Autodesk Inventor part; units mm, degrees
(part 6 of 6)
  line L4439 (-10.0121, 28.4168) -> (-10.0047, 28.6447)
  line L4440 (-10.0047, 28.6447) -> (-9.9918, 28.8863)
  line L4441 (-9.9918, 28.8863) -> (-9.973, 29.1388)
  line L4442 (-9.973, 29.1388) -> (-9.9523, 29.359)
  arc A136 (-9.2052, 29.6018) -> (-9.9523, 29.359) centre (0, 0) ccw
  line L4443 (-9.2052, 29.6018) -> (-9.059, 29.4358)
  line L4444 (-9.059, 29.4358) -> (-8.8954, 29.2425)
  line L4445 (-8.8954, 29.2425) -> (-8.7429, 29.0547)
  line L4446 (-8.7429, 29.0547) -> (-8.603, 28.8746)
  line L4447 (-8.603, 28.8746) -> (-8.4737, 28.7009)
  line L4448 (-8.4737, 28.7009) -> (-8.3547, 28.5338)
  line L4449 (-8.3547, 28.5338) -> (-8.2472, 28.3759)
  line L4450 (-8.2472, 28.3759) -> (-8.1494, 28.2257)
  line L4451 (-8.1494, 28.2257) -> (-7.9652, 27.9266)
  line L4452 (-7.9652, 27.9266) -> (-7.9351, 27.8907)
  line L4453 (-7.9351, 27.8907) -> (-7.9073, 27.8683)
  line L4454 (-7.9073, 27.8683) -> (-7.8823, 27.8592)
  line L4455 (-7.8823, 27.8592) -> (-7.8657, 27.861)
  line L4456 (-7.8657, 27.861) -> (-7.4928, 27.9636)
  line L4457 (-7.4928, 27.9636) -> (-7.1186, 28.0612)
  line L4458 (-7.1186, 28.0612) -> (-7.1033, 28.0679)
  line L4459 (-7.1033, 28.0679) -> (-7.0862, 28.0883)
  line L4460 (-7.0862, 28.0883) -> (-7.0733, 28.1216)
  line L4461 (-7.0733, 28.1216) -> (-7.0652, 28.1677)
  line L4462 (-7.0652, 28.1677) -> (-7.0553, 28.5189)
  line L4463 (-7.0553, 28.5189) -> (-7.0457, 28.6979)
  line L4464 (-7.0457, 28.6979) -> (-7.0315, 28.8883)
  line L4465 (-7.0315, 28.8883) -> (-7.012, 29.0926)
  line L4466 (-7.012, 29.0926) -> (-6.9869, 29.3077)
  line L4467 (-6.9869, 29.3077) -> (-6.9557, 29.5336)
  line L4468 (-6.9557, 29.5336) -> (-6.9177, 29.7725)
  line L4469 (-6.9177, 29.7725) -> (-6.8726, 30.0216)
  line L4470 (-6.8726, 30.0216) -> (-6.829, 30.2385)
  arc A137 (-6.0605, 30.4018) -> (-6.829, 30.2385) centre (0, 0) ccw
  line L4471 (-6.0605, 30.4018) -> (-5.9325, 30.2214)
  line L4472 (-5.9325, 30.2214) -> (-5.79, 30.0122)
  line L4473 (-5.79, 30.0122) -> (-5.658, 29.8094)
  line L4474 (-5.658, 29.8094) -> (-5.5376, 29.6157)
  line L4475 (-5.5376, 29.6157) -> (-5.4272, 29.4294)
  line L4476 (-5.4272, 29.4294) -> (-5.3263, 29.2508)
  line L4477 (-5.3263, 29.2508) -> (-5.2359, 29.0826)
  line L4478 (-5.2359, 29.0826) -> (-5.1544, 28.9229)
  line L4479 (-5.1544, 28.9229) -> (-5.0025, 28.6062)
  line L4480 (-5.0025, 28.6062) -> (-4.9763, 28.5674)
  line L4481 (-4.9763, 28.5674) -> (-4.951, 28.5421)
  line L4482 (-4.951, 28.5421) -> (-4.927, 28.5305)
  line L4483 (-4.927, 28.5305) -> (-4.9104, 28.5306)
  line L4484 (-4.9104, 28.5306) -> (-4.5288, 28.5936)
  line L4485 (-4.5288, 28.5936) -> (-4.1464, 28.6516)
  line L4486 (-4.1464, 28.6516) -> (-4.1305, 28.6567)
  line L4487 (-4.1305, 28.6567) -> (-4.1114, 28.6751)
  line L4488 (-4.1114, 28.6751) -> (-4.0951, 28.7069)
  line L4489 (-4.0951, 28.7069) -> (-4.0822, 28.7519)
  line L4490 (-4.0822, 28.7519) -> (-4.0356, 29.1001)
  line L4491 (-4.0356, 29.1001) -> (-4.0074, 29.2771)
  line L4492 (-4.0074, 29.2771) -> (-3.9734, 29.465)
  line L4493 (-3.9734, 29.465) -> (-3.9326, 29.6661)
  line L4494 (-3.9326, 29.6661) -> (-3.8852, 29.8774)
  line L4495 (-3.8852, 29.8774) -> (-3.8305, 30.0989)
  line L4496 (-3.8305, 30.0989) -> (-3.7677, 30.3325)
  line L4497 (-3.7677, 30.3325) -> (-3.6968, 30.5755)
  line L4498 (-3.6968, 30.5755) -> (-3.6308, 30.7866)
  arc A138 (-2.8495, 30.8688) -> (-3.6308, 30.7866) centre (0, 0) ccw
  line L4499 (-2.8495, 30.8688) -> (-2.741, 30.676)
  line L4500 (-2.741, 30.676) -> (-2.6211, 30.453)
  line L4501 (-2.6211, 30.453) -> (-2.5111, 30.2376)
  line L4502 (-2.5111, 30.2376) -> (-2.4116, 30.0323)
  line L4503 (-2.4116, 30.0323) -> (-2.3213, 29.8355)
  line L4504 (-2.3213, 29.8355) -> (-2.2396, 29.6473)
  line L4505 (-2.2396, 29.6473) -> (-2.1673, 29.4705)
  line L4506 (-2.1673, 29.4705) -> (-2.1029, 29.3033)
  line L4507 (-2.1029, 29.3033) -> (-1.9849, 28.9724)
  line L4508 (-1.9849, 28.9724) -> (-1.9629, 28.931)
  line L4509 (-1.9629, 28.931) -> (-1.9404, 28.9033)
  line L4510 (-1.9404, 28.9033) -> (-1.9178, 28.8892)
  line L4511 (-1.9178, 28.8892) -> (-1.9012, 28.8876)
  line L4512 (-1.9012, 28.8876) -> (-1.5151, 28.9103)
  line L4513 (-1.5151, 28.9103) -> (-1.1288, 28.9281)
  line L4514 (-1.1288, 28.9281) -> (-1.1124, 28.9314)
  line L4515 (-1.1124, 28.9314) -> (-1.0915, 28.9478)
  line L4516 (-1.0915, 28.9478) -> (-1.0719, 28.9777)
  line L4517 (-1.0719, 28.9777) -> (-1.0544, 29.0211)
  line L4518 (-1.0544, 29.0211) -> (-0.9717, 29.3626)
  line L4519 (-0.9717, 29.3626) -> (-0.9251, 29.5356)
  line L4520 (-0.9251, 29.5356) -> (-0.8717, 29.719)
  line L4521 (-0.8717, 29.719) -> (-0.8101, 29.9147)
  line L4522 (-0.8101, 29.9147) -> (-0.7408, 30.1199)
  line L4523 (-0.7408, 30.1199) -> (-0.6634, 30.3344)
  line L4524 (-0.6634, 30.3344) -> (-0.5765, 30.5601)
  line L4525 (-0.5765, 30.5601) -> (-0.4805, 30.7945)
  line L4526 (-0.4805, 30.7945) -> (-0.3928, 30.9975)
  arc A139 (0.3928, 30.9975) -> (-0.3928, 30.9975) centre (0, 0) ccw
  line L4527 (0.3928, 30.9975) -> (0.4805, 30.7945)
  line L4528 (0.4805, 30.7945) -> (0.5765, 30.5601)
  line L4529 (0.5765, 30.5601) -> (0.6634, 30.3344)
  line L4530 (0.6634, 30.3344) -> (0.7408, 30.1199)
  line L4531 (0.7408, 30.1199) -> (0.8101, 29.9147)
  line L4532 (0.8101, 29.9147) -> (0.8717, 29.719)
  line L4533 (0.8717, 29.719) -> (0.9251, 29.5356)
  line L4534 (0.9251, 29.5356) -> (0.9717, 29.3626)
  line L4535 (0.9717, 29.3626) -> (1.0544, 29.0211)
  line L4536 (1.0544, 29.0211) -> (1.0719, 28.9777)
  line L4537 (1.0719, 28.9777) -> (1.0915, 28.9478)
  line L4538 (1.0915, 28.9478) -> (1.1124, 28.9314)
  line L4539 (1.1124, 28.9314) -> (1.1288, 28.9281)
  line L4540 (1.1288, 28.9281) -> (1.5151, 28.9103)
  line L4541 (1.5151, 28.9103) -> (1.9012, 28.8876)
  line L4542 (1.9012, 28.8876) -> (1.9178, 28.8892)
  line L4543 (1.9178, 28.8892) -> (1.9404, 28.9033)
  line L4544 (1.9404, 28.9033) -> (1.9629, 28.931)
  line L4545 (1.9629, 28.931) -> (1.9849, 28.9724)
  line L4546 (1.9849, 28.9724) -> (2.1029, 29.3033)
  line L4547 (2.1029, 29.3033) -> (2.1673, 29.4705)
  line L4548 (2.1673, 29.4705) -> (2.2396, 29.6473)
  line L4549 (2.2396, 29.6473) -> (2.3213, 29.8355)
  line L4550 (2.3213, 29.8355) -> (2.4116, 30.0323)
  line L4551 (2.4116, 30.0323) -> (2.5111, 30.2376)
  line L4552 (2.5111, 30.2376) -> (2.6211, 30.453)
  line L4553 (2.6211, 30.453) -> (2.741, 30.676)
  line L4554 (2.741, 30.676) -> (2.8495, 30.8688)
  arc A140 (3.6308, 30.7866) -> (2.8495, 30.8688) centre (0, 0) ccw
  line L4555 (3.6308, 30.7866) -> (3.6968, 30.5755)
  line L4556 (3.6968, 30.5755) -> (3.7677, 30.3325)
  line L4557 (3.7677, 30.3325) -> (3.8305, 30.0989)
  line L4558 (3.8305, 30.0989) -> (3.8852, 29.8774)
  line L4559 (3.8852, 29.8774) -> (3.9326, 29.6661)
  line L4560 (3.9326, 29.6661) -> (3.9734, 29.465)
  line L4561 (3.9734, 29.465) -> (4.0074, 29.2771)
  line L4562 (4.0074, 29.2771) -> (4.0356, 29.1001)
  line L4563 (4.0356, 29.1001) -> (4.0822, 28.7519)
  line L4564 (4.0822, 28.7519) -> (4.0951, 28.7069)
  line L4565 (4.0951, 28.7069) -> (4.1114, 28.6751)
  line L4566 (4.1114, 28.6751) -> (4.1305, 28.6567)
  line L4567 (4.1305, 28.6567) -> (4.1464, 28.6516)
  line L4568 (4.1464, 28.6516) -> (4.5288, 28.5936)
  line L4569 (4.5288, 28.5936) -> (4.9104, 28.5306)
  line L4570 (4.9104, 28.5306) -> (4.927, 28.5305)
  line L4571 (4.927, 28.5305) -> (4.951, 28.5421)
  line L4572 (4.951, 28.5421) -> (4.9763, 28.5674)
  line L4573 (4.9763, 28.5674) -> (5.0025, 28.6062)
  line L4574 (5.0025, 28.6062) -> (5.1544, 28.9229)
  line L4575 (5.1544, 28.9229) -> (5.2359, 29.0826)
  line L4576 (5.2359, 29.0826) -> (5.3263, 29.2508)
  line L4577 (5.3263, 29.2508) -> (5.4272, 29.4294)
  line L4578 (5.4272, 29.4294) -> (5.5376, 29.6157)
  line L4579 (5.5376, 29.6157) -> (5.658, 29.8094)
  line L4580 (5.658, 29.8094) -> (5.79, 30.0122)
  line L4581 (5.79, 30.0122) -> (5.9325, 30.2214)
  line L4582 (5.9325, 30.2214) -> (6.0605, 30.4018)
  arc A141 (6.829, 30.2385) -> (6.0605, 30.4018) centre (0, 0) ccw
  line L4583 (6.829, 30.2385) -> (6.8726, 30.0216)
  line L4584 (6.8726, 30.0216) -> (6.9177, 29.7725)
  line L4585 (6.9177, 29.7725) -> (6.9557, 29.5336)
  line L4586 (6.9557, 29.5336) -> (6.9869, 29.3077)
  line L4587 (6.9869, 29.3077) -> (7.012, 29.0926)
  line L4588 (7.012, 29.0926) -> (7.0315, 28.8883)
  line L4589 (7.0315, 28.8883) -> (7.0457, 28.6979)
  line L4590 (7.0457, 28.6979) -> (7.0553, 28.5189)
  line L4591 (7.0553, 28.5189) -> (7.0652, 28.1677)
  line L4592 (7.0652, 28.1677) -> (7.0733, 28.1216)
  line L4593 (7.0733, 28.1216) -> (7.0862, 28.0883)
  line L4594 (7.0862, 28.0883) -> (7.1033, 28.0679)
  line L4595 (7.1033, 28.0679) -> (7.1186, 28.0612)
  line L4596 (7.1186, 28.0612) -> (7.4928, 27.9636)
  line L4597 (7.4928, 27.9636) -> (7.8657, 27.861)
  line L4598 (7.8657, 27.861) -> (7.8823, 27.8592)
  line L4599 (7.8823, 27.8592) -> (7.9073, 27.8683)
  line L4600 (7.9073, 27.8683) -> (7.9351, 27.8907)
  line L4601 (7.9351, 27.8907) -> (7.9652, 27.9266)
  line L4602 (7.9652, 27.9266) -> (8.1494, 28.2257)
  line L4603 (8.1494, 28.2257) -> (8.2472, 28.3759)
  line L4604 (8.2472, 28.3759) -> (8.3547, 28.5338)
  line L4605 (8.3547, 28.5338) -> (8.4737, 28.7009)
  line L4606 (8.4737, 28.7009) -> (8.603, 28.8746)
  line L4607 (8.603, 28.8746) -> (8.7429, 29.0547)
  line L4608 (8.7429, 29.0547) -> (8.8954, 29.2425)
  line L4609 (8.8954, 29.2425) -> (9.059, 29.4358)
  line L4610 (9.059, 29.4358) -> (9.2052, 29.6018)
  arc A142 (9.9523, 29.359) -> (9.2052, 29.6018) centre (0, 0) ccw
  line L4611 (9.9523, 29.359) -> (9.973, 29.1388)
  line L4612 (9.973, 29.1388) -> (9.9918, 28.8863)
  line L4613 (9.9918, 28.8863) -> (10.0047, 28.6447)
  line L4614 (10.0047, 28.6447) -> (10.0121, 28.4168)
  line L4615 (10.0121, 28.4168) -> (10.0146, 28.2002)
  line L4616 (10.0146, 28.2002) -> (10.0127, 27.995)
  line L4617 (10.0127, 27.995) -> (10.0069, 27.8042)
  line L4618 (10.0069, 27.8042) -> (9.9977, 27.6252)
  line L4619 (9.9977, 27.6252) -> (9.9708, 27.2749)
  line L4620 (9.9708, 27.2749) -> (9.9741, 27.2282)
  line L4621 (9.9741, 27.2282) -> (9.9834, 27.1937)
  line L4622 (9.9834, 27.1937) -> (9.9983, 27.1717)
  line L4623 (9.9983, 27.1717) -> (10.0128, 27.1634)
  line L4624 (10.0128, 27.1634) -> (10.3748, 27.0272)
  line L4625 (10.3748, 27.0272) -> (10.7349, 26.8862)
  line L4626 (10.7349, 26.8862) -> (10.7512, 26.8826)
  line L4627 (10.7512, 26.8826) -> (10.777, 26.8891)
  line L4628 (10.777, 26.8891) -> (10.807, 26.9085)
  line L4629 (10.807, 26.9085) -> (10.8407, 26.941)
  line L4630 (10.8407, 26.941) -> (11.0551, 27.2193)
  line L4631 (11.0551, 27.2193) -> (11.1681, 27.3584)
  line L4632 (11.1681, 27.3584) -> (11.2915, 27.5042)
  line L4633 (11.2915, 27.5042) -> (11.4273, 27.6579)
  line L4634 (11.4273, 27.6579) -> (11.5741, 27.8172)
  line L4635 (11.5741, 27.8172) -> (11.7321, 27.9817)
  line L4636 (11.7321, 27.9817) -> (11.9033, 28.1525)
  line L4637 (11.9033, 28.1525) -> (12.0862, 28.3276)
  line L4638 (12.0862, 28.3276) -> (12.249, 28.4774)
  arc A143 (12.9667, 28.1579) -> (12.249, 28.4774) centre (0, 0) ccw
  line L4639 (12.9667, 28.1579) -> (12.9642, 27.9367)
  line L4640 (12.9642, 27.9367) -> (12.9565, 27.6836)
  line L4641 (12.9565, 27.6836) -> (12.9441, 27.442)
  line L4642 (12.9441, 27.442) -> (12.9276, 27.2145)
  line L4643 (12.9276, 27.2145) -> (12.9075, 26.9989)
  line L4644 (12.9075, 26.9989) -> (12.8841, 26.7951)
  line L4645 (12.8841, 26.7951) -> (12.8584, 26.6059)
  line L4646 (12.8584, 26.6059) -> (12.8305, 26.4288)
  line L4647 (12.8305, 26.4288) -> (12.7672, 26.0833)
  line L4648 (12.7672, 26.0833) -> (12.7656, 26.0365)
  line L4649 (12.7656, 26.0365) -> (12.7712, 26.0012)
  line L4650 (12.7712, 26.0012) -> (12.7837, 25.9777)
  line L4651 (12.7837, 25.9777) -> (12.7973, 25.968)
  line L4652 (12.7973, 25.968) -> (13.143, 25.7946)
  line L4653 (13.143, 25.7946) -> (13.4865, 25.6168)
  line L4654 (13.4865, 25.6168) -> (13.5023, 25.6116)
  line L4655 (13.5023, 25.6116) -> (13.5287, 25.6153)
  line L4656 (13.5287, 25.6153) -> (13.5605, 25.6314)
  line L4657 (13.5605, 25.6314) -> (13.5974, 25.6603)
  line L4658 (13.5974, 25.6603) -> (13.8398, 25.9146)
  line L4659 (13.8398, 25.9146) -> (13.9666, 26.0412)
  line L4660 (13.9666, 26.0412) -> (14.1046, 26.1732)
  line L4661 (14.1046, 26.1732) -> (14.2558, 26.312)
  line L4662 (14.2558, 26.312) -> (14.4184, 26.455)
  line L4663 (14.4184, 26.455) -> (14.5927, 26.602)
  line L4664 (14.5927, 26.602) -> (14.7808, 26.7541)
  line L4665 (14.7808, 26.7541) -> (14.9811, 26.9091)
  line L4666 (14.9811, 26.9091) -> (15.1586, 27.041)
  arc A144 (15.8389, 26.6482) -> (15.1586, 27.041) centre (0, 0) ccw
  line L4667 (15.8389, 26.6482) -> (15.8134, 26.4285)
  line L4668 (15.8134, 26.4285) -> (15.7793, 26.1776)
  line L4669 (15.7793, 26.1776) -> (15.7417, 25.9387)
  line L4670 (15.7417, 25.9387) -> (15.7015, 25.7142)
  line L4671 (15.7015, 25.7142) -> (15.6589, 25.5018)
  line L4672 (15.6589, 25.5018) -> (15.6144, 25.3015)
  line L4673 (15.6144, 25.3015) -> (15.569, 25.1161)
  line L4674 (15.569, 25.1161) -> (15.5228, 24.9429)
  line L4675 (15.5228, 24.9429) -> (15.4237, 24.6058)
  line L4676 (15.4237, 24.6058) -> (15.4172, 24.5595)
  line L4677 (15.4172, 24.5595) -> (15.4191, 24.5238)
  line L4678 (15.4191, 24.5238) -> (15.4291, 24.4991)
  line L4679 (15.4291, 24.4991) -> (15.4416, 24.488)
  line L4680 (15.4416, 24.488) -> (15.7673, 24.2795)
  line L4681 (15.7673, 24.2795) -> (16.0903, 24.0668)
  line L4682 (16.0903, 24.0668) -> (16.1055, 24.0599)
  line L4683 (16.1055, 24.0599) -> (16.1321, 24.0608)
  line L4684 (16.1321, 24.0608) -> (16.1655, 24.0735)
  line L4685 (16.1655, 24.0735) -> (16.2052, 24.0984)
  line L4686 (16.2052, 24.0984) -> (16.4728, 24.326)
  line L4687 (16.4728, 24.326) -> (16.6122, 24.4386)
  line L4688 (16.6122, 24.4386) -> (16.7632, 24.5555)
  line L4689 (16.7632, 24.5555) -> (16.928, 24.6777)
  line L4690 (16.928, 24.6777) -> (17.1047, 24.8029)
  line L4691 (17.1047, 24.8029) -> (17.2934, 24.931)
  line L4692 (17.2934, 24.931) -> (17.4964, 25.0625)
  line L4693 (17.4964, 25.0625) -> (17.7118, 25.1957)
  line L4694 (17.7118, 25.1957) -> (17.9021, 25.3084)
  arc A145 (18.5377, 24.8466) -> (17.9021, 25.3084) centre (0, 0) ccw
  line L4695 (18.5377, 24.8466) -> (18.4893, 24.6308)
  line L4696 (18.4893, 24.6308) -> (18.4292, 24.3848)
  line L4697 (18.4292, 24.3848) -> (18.3668, 24.1511)
  line L4698 (18.3668, 24.1511) -> (18.3034, 23.932)
  line L4699 (18.3034, 23.932) -> (18.2388, 23.7253)
  line L4700 (18.2388, 23.7253) -> (18.1736, 23.5308)
  line L4701 (18.1736, 23.5308) -> (18.1091, 23.3511)
  line L4702 (18.1091, 23.3511) -> (18.045, 23.1837)
  line L4703 (18.045, 23.1837) -> (17.9112, 22.8588)
  line L4704 (17.9112, 22.8588) -> (17.8999, 22.8134)
  line L4705 (17.8999, 22.8134) -> (17.8981, 22.7777)
  line L4706 (17.8981, 22.7777) -> (17.9055, 22.7521)
  line L4707 (17.9055, 22.7521) -> (17.9167, 22.7398)
  line L4708 (17.9167, 22.7398) -> (18.2188, 22.4984)
  line L4709 (18.2188, 22.4984) -> (18.5178, 22.2531)
  line L4710 (18.5178, 22.2531) -> (18.5322, 22.2446)
  line L4711 (18.5322, 22.2446) -> (18.5587, 22.2427)
  line L4712 (18.5587, 22.2427) -> (18.5933, 22.2519)
  line L4713 (18.5933, 22.2519) -> (18.6353, 22.2724)
  line L4714 (18.6353, 22.2724) -> (18.9253, 22.4708)
  line L4715 (18.9253, 22.4708) -> (19.0757, 22.5683)
  line L4716 (19.0757, 22.5683) -> (19.2381, 22.6688)
  line L4717 (19.2381, 22.6688) -> (19.4148, 22.773)
  line L4718 (19.4148, 22.773) -> (19.6036, 22.8791)
  line L4719 (19.6036, 22.8791) -> (19.8047, 22.9867)
  line L4720 (19.8047, 22.9867) -> (20.0203, 23.0963)
  line L4721 (20.0203, 23.0963) -> (20.2484, 23.2063)
  line L4722 (20.2484, 23.2063) -> (20.4495, 23.2985)
  arc A146 (21.0333, 22.7728) -> (20.4495, 23.2985) centre (0, 0) ccw
  line L4723 (21.0333, 22.7728) -> (20.9626, 22.5632)
  line L4724 (20.9626, 22.5632) -> (20.8771, 22.3249)
  line L4725 (20.8771, 22.3249) -> (20.7906, 22.099)
  line L4726 (20.7906, 22.099) -> (20.7047, 21.8877)
  line L4727 (20.7047, 21.8877) -> (20.6189, 21.6889)
  line L4728 (20.6189, 21.6889) -> (20.5336, 21.5022)
  line L4729 (20.5336, 21.5022) -> (20.4507, 21.3302)
  line L4730 (20.4507, 21.3302) -> (20.3695, 21.1705)
  line L4731 (20.3695, 21.1705) -> (20.2025, 20.8614)
  line L4732 (20.2025, 20.8614) -> (20.1865, 20.8174)
  line L4733 (20.1865, 20.8174) -> (20.181, 20.7821)
  line L4734 (20.181, 20.7821) -> (20.1856, 20.7559)
  line L4735 (20.1856, 20.7559) -> (20.1955, 20.7424)
  line L4736 (20.1955, 20.7424) -> (20.4707, 20.4707)
  line L4737 (20.4707, 20.4707) -> (20.7424, 20.1955)
  line L4738 (20.7424, 20.1955) -> (20.7559, 20.1856)
  line L4739 (20.7559, 20.1856) -> (20.7821, 20.181)
  line L4740 (20.7821, 20.181) -> (20.8174, 20.1865)
  line L4741 (20.8174, 20.1865) -> (20.8614, 20.2025)
  line L4742 (20.8614, 20.2025) -> (21.1705, 20.3695)
  line L4743 (21.1705, 20.3695) -> (21.3302, 20.4507)
  line L4744 (21.3302, 20.4507) -> (21.5022, 20.5336)
  line L4745 (21.5022, 20.5336) -> (21.6889, 20.6189)
  line L4746 (21.6889, 20.6189) -> (21.8877, 20.7047)
  line L4747 (21.8877, 20.7047) -> (22.099, 20.7906)
  line L4748 (22.099, 20.7906) -> (22.3249, 20.8771)
  line L4749 (22.3249, 20.8771) -> (22.5632, 20.9626)
  line L4750 (22.5632, 20.9626) -> (22.7728, 21.0333)
  arc A147 (23.2985, 20.4495) -> (22.7728, 21.0333) centre (0, 0) ccw
  line L4751 (23.2985, 20.4495) -> (23.2063, 20.2484)
  line L4752 (23.2063, 20.2484) -> (23.0963, 20.0203)
  line L4753 (23.0963, 20.0203) -> (22.9867, 19.8047)
  line L4754 (22.9867, 19.8047) -> (22.8791, 19.6036)
  line L4755 (22.8791, 19.6036) -> (22.773, 19.4148)
  line L4756 (22.773, 19.4148) -> (22.6688, 19.2381)
  line L4757 (22.6688, 19.2381) -> (22.5683, 19.0757)
  line L4758 (22.5683, 19.0757) -> (22.4708, 18.9253)
  line L4759 (22.4708, 18.9253) -> (22.2724, 18.6353)
  line L4760 (22.2724, 18.6353) -> (22.2519, 18.5933)
  line L4761 (22.2519, 18.5933) -> (22.2427, 18.5587)
  line L4762 (22.2427, 18.5587) -> (22.2446, 18.5322)
  line L4763 (22.2446, 18.5322) -> (22.2531, 18.5178)
  line L4764 (22.2531, 18.5178) -> (22.4984, 18.2188)
  line L4765 (22.4984, 18.2188) -> (22.7398, 17.9167)
  line L4766 (22.7398, 17.9167) -> (22.7521, 17.9055)
  line L4767 (22.7521, 17.9055) -> (22.7777, 17.8981)
  line L4768 (22.7777, 17.8981) -> (22.8134, 17.8999)
  line L4769 (22.8134, 17.8999) -> (22.8588, 17.9112)
  line L4770 (22.8588, 17.9112) -> (23.1837, 18.045)
  line L4771 (23.1837, 18.045) -> (23.3511, 18.1091)
  line L4772 (23.3511, 18.1091) -> (23.5308, 18.1736)
  line L4773 (23.5308, 18.1736) -> (23.7253, 18.2388)
  line L4774 (23.7253, 18.2388) -> (23.932, 18.3034)
  line L4775 (23.932, 18.3034) -> (24.1511, 18.3668)
  line L4776 (24.1511, 18.3668) -> (24.3848, 18.4292)
  line L4777 (24.3848, 18.4292) -> (24.6308, 18.4893)
  line L4778 (24.6308, 18.4893) -> (24.8466, 18.5377)
  arc A148 (25.3084, 17.9021) -> (24.8466, 18.5377) centre (0, 0) ccw
  line L4779 (25.3084, 17.9021) -> (25.1957, 17.7118)
  line L4780 (25.1957, 17.7118) -> (25.0625, 17.4964)
  line L4781 (25.0625, 17.4964) -> (24.931, 17.2934)
  line L4782 (24.931, 17.2934) -> (24.8029, 17.1047)
  line L4783 (24.8029, 17.1047) -> (24.6777, 16.928)
  line L4784 (24.6777, 16.928) -> (24.5555, 16.7632)
  line L4785 (24.5555, 16.7632) -> (24.4386, 16.6122)
  line L4786 (24.4386, 16.6122) -> (24.326, 16.4728)
  line L4787 (24.326, 16.4728) -> (24.0984, 16.2052)
  line L4788 (24.0984, 16.2052) -> (24.0735, 16.1655)
  line L4789 (24.0735, 16.1655) -> (24.0608, 16.1321)
  line L4790 (24.0608, 16.1321) -> (24.0599, 16.1055)
  line L4791 (24.0599, 16.1055) -> (24.0668, 16.0903)
  line L4792 (24.0668, 16.0903) -> (24.2795, 15.7673)
  line L4793 (24.2795, 15.7673) -> (24.488, 15.4416)
  line L4794 (24.488, 15.4416) -> (24.4991, 15.4291)
  line L4795 (24.4991, 15.4291) -> (24.5238, 15.4191)
  line L4796 (24.5238, 15.4191) -> (24.5595, 15.4172)
  line L4797 (24.5595, 15.4172) -> (24.6058, 15.4237)
  line L4798 (24.6058, 15.4237) -> (24.9429, 15.5228)
  line L4799 (24.9429, 15.5228) -> (25.1161, 15.569)
  line L4800 (25.1161, 15.569) -> (25.3015, 15.6144)
  line L4801 (25.3015, 15.6144) -> (25.5018, 15.6589)
  line L4802 (25.5018, 15.6589) -> (25.7142, 15.7015)
  line L4803 (25.7142, 15.7015) -> (25.9387, 15.7417)
  line L4804 (25.9387, 15.7417) -> (26.1776, 15.7793)
  line L4805 (26.1776, 15.7793) -> (26.4285, 15.8134)
  line L4806 (26.4285, 15.8134) -> (26.6482, 15.8389)
  arc A149 (27.041, 15.1586) -> (26.6482, 15.8389) centre (0, 0) ccw
  line L4807 (27.041, 15.1586) -> (26.9091, 14.9811)
  line L4808 (26.9091, 14.9811) -> (26.7541, 14.7808)
  line L4809 (26.7541, 14.7808) -> (26.602, 14.5927)
  line L4810 (26.602, 14.5927) -> (26.455, 14.4184)
  line L4811 (26.455, 14.4184) -> (26.312, 14.2558)
  line L4812 (26.312, 14.2558) -> (26.1732, 14.1046)
  line L4813 (26.1732, 14.1046) -> (26.0412, 13.9666)
  line L4814 (26.0412, 13.9666) -> (25.9146, 13.8398)
  line L4815 (25.9146, 13.8398) -> (25.6603, 13.5974)
  line L4816 (25.6603, 13.5974) -> (25.6314, 13.5605)
  line L4817 (25.6314, 13.5605) -> (25.6153, 13.5287)
  line L4818 (25.6153, 13.5287) -> (25.6116, 13.5023)
  line L4819 (25.6116, 13.5023) -> (25.6168, 13.4865)
  line L4820 (25.6168, 13.4865) -> (25.7946, 13.143)
  line L4821 (25.7946, 13.143) -> (25.968, 12.7973)
  line L4822 (25.968, 12.7973) -> (25.9777, 12.7837)
  line L4823 (25.9777, 12.7837) -> (26.0012, 12.7712)
  line L4824 (26.0012, 12.7712) -> (26.0365, 12.7656)
  line L4825 (26.0365, 12.7656) -> (26.0833, 12.7672)
  line L4826 (26.0833, 12.7672) -> (26.4288, 12.8305)
  line L4827 (26.4288, 12.8305) -> (26.6059, 12.8584)
  line L4828 (26.6059, 12.8584) -> (26.7951, 12.8841)
  line L4829 (26.7951, 12.8841) -> (26.9989, 12.9075)
  line L4830 (26.9989, 12.9075) -> (27.2145, 12.9276)
  line L4831 (27.2145, 12.9276) -> (27.442, 12.9441)
  line L4832 (27.442, 12.9441) -> (27.6836, 12.9565)
  line L4833 (27.6836, 12.9565) -> (27.9367, 12.9642)
  line L4834 (27.9367, 12.9642) -> (28.1579, 12.9667)
  arc A150 (28.4774, 12.249) -> (28.1579, 12.9667) centre (0, 0) ccw
  line L4835 (28.4774, 12.249) -> (28.3276, 12.0862)
  line L4836 (28.3276, 12.0862) -> (28.1525, 11.9033)
  line L4837 (28.1525, 11.9033) -> (27.9817, 11.7321)
  line L4838 (27.9817, 11.7321) -> (27.8172, 11.5741)
  line L4839 (27.8172, 11.5741) -> (27.6579, 11.4273)
  line L4840 (27.6579, 11.4273) -> (27.5042, 11.2915)
  line L4841 (27.5042, 11.2915) -> (27.3584, 11.1681)
  line L4842 (27.3584, 11.1681) -> (27.2193, 11.0551)
  line L4843 (27.2193, 11.0551) -> (26.941, 10.8407)
  line L4844 (26.941, 10.8407) -> (26.9085, 10.807)
  line L4845 (26.9085, 10.807) -> (26.8891, 10.777)
  line L4846 (26.8891, 10.777) -> (26.8826, 10.7512)
  line L4847 (26.8826, 10.7512) -> (26.8862, 10.7349)
  line L4848 (26.8862, 10.7349) -> (27.0272, 10.3748)
  line L4849 (27.0272, 10.3748) -> (27.1634, 10.0128)
  line L4850 (27.1634, 10.0128) -> (27.1717, 9.9983)
  line L4851 (27.1717, 9.9983) -> (27.1937, 9.9834)
  line L4852 (27.1937, 9.9834) -> (27.2282, 9.9741)
  line L4853 (27.2282, 9.9741) -> (27.2749, 9.9708)
  line L4854 (27.2749, 9.9708) -> (27.6252, 9.9977)
  line L4855 (27.6252, 9.9977) -> (27.8042, 10.0069)
  line L4856 (27.8042, 10.0069) -> (27.995, 10.0127)
  line L4857 (27.995, 10.0127) -> (28.2002, 10.0146)
  line L4858 (28.2002, 10.0146) -> (28.4168, 10.0121)
  line L4859 (28.4168, 10.0121) -> (28.6447, 10.0047)
  line L4860 (28.6447, 10.0047) -> (28.8863, 9.9918)
  line L4861 (28.8863, 9.9918) -> (29.1388, 9.973)
  line L4862 (29.1388, 9.973) -> (29.359, 9.9523)
  arc A151 (29.6018, 9.2052) -> (29.359, 9.9523) centre (0, 0) ccw
  line L4863 (29.6018, 9.2052) -> (29.4358, 9.059)
  line L4864 (29.4358, 9.059) -> (29.2425, 8.8954)
  line L4865 (29.2425, 8.8954) -> (29.0547, 8.7429)
  line L4866 (29.0547, 8.7429) -> (28.8746, 8.603)
  line L4867 (28.8746, 8.603) -> (28.7009, 8.4737)
  line L4868 (28.7009, 8.4737) -> (28.5338, 8.3547)
  line L4869 (28.5338, 8.3547) -> (28.3759, 8.2472)
  line L4870 (28.3759, 8.2472) -> (28.2257, 8.1494)
  line L4871 (28.2257, 8.1494) -> (27.9266, 7.9652)
  line L4872 (27.9266, 7.9652) -> (27.8907, 7.9351)
  line L4873 (27.8907, 7.9351) -> (27.8683, 7.9073)
  line L4874 (27.8683, 7.9073) -> (27.8592, 7.8823)
  line L4875 (27.8592, 7.8823) -> (27.861, 7.8657)
  line L4876 (27.861, 7.8657) -> (27.9636, 7.4928)
  line L4877 (27.9636, 7.4928) -> (28.0612, 7.1186)
  line L4878 (28.0612, 7.1186) -> (28.0679, 7.1033)
  line L4879 (28.0679, 7.1033) -> (28.0883, 7.0862)
  line L4880 (28.0883, 7.0862) -> (28.1216, 7.0733)
  line L4881 (28.1216, 7.0733) -> (28.1677, 7.0652)
  line L4882 (28.1677, 7.0652) -> (28.5189, 7.0553)
  line L4883 (28.5189, 7.0553) -> (28.6979, 7.0457)
  line L4884 (28.6979, 7.0457) -> (28.8883, 7.0315)
  line L4885 (28.8883, 7.0315) -> (29.0926, 7.012)
  line L4886 (29.0926, 7.012) -> (29.3077, 6.9869)
  line L4887 (29.3077, 6.9869) -> (29.5336, 6.9557)
  line L4888 (29.5336, 6.9557) -> (29.7725, 6.9177)
  line L4889 (29.7725, 6.9177) -> (30.0216, 6.8726)
  line L4890 (30.0216, 6.8726) -> (30.2385, 6.829)
  arc A152 (30.4018, 6.0605) -> (30.2385, 6.829) centre (0, 0) ccw
  line L4891 (30.4018, 6.0605) -> (30.2214, 5.9325)
  line L4892 (30.2214, 5.9325) -> (30.0122, 5.79)
  line L4893 (30.0122, 5.79) -> (29.8094, 5.658)
  line L4894 (29.8094, 5.658) -> (29.6157, 5.5376)
  line L4895 (29.6157, 5.5376) -> (29.4294, 5.4272)
  line L4896 (29.4294, 5.4272) -> (29.2508, 5.3263)
  line L4897 (29.2508, 5.3263) -> (29.0826, 5.2359)
  line L4898 (29.0826, 5.2359) -> (28.9229, 5.1544)
  line L4899 (28.9229, 5.1544) -> (28.6062, 5.0025)
  line L4900 (28.6062, 5.0025) -> (28.5674, 4.9763)
  line L4901 (28.5674, 4.9763) -> (28.5421, 4.951)
  line L4902 (28.5421, 4.951) -> (28.5305, 4.927)
  line L4903 (28.5305, 4.927) -> (28.5306, 4.9104)
  line L4904 (28.5306, 4.9104) -> (28.5936, 4.5288)
  line L4905 (28.5936, 4.5288) -> (28.6516, 4.1464)
  line L4906 (28.6516, 4.1464) -> (28.6567, 4.1305)
  line L4907 (28.6567, 4.1305) -> (28.6751, 4.1114)
  line L4908 (28.6751, 4.1114) -> (28.7069, 4.0951)
  line L4909 (28.7069, 4.0951) -> (28.7519, 4.0822)
  line L4910 (28.7519, 4.0822) -> (29.1001, 4.0356)
  line L4911 (29.1001, 4.0356) -> (29.2771, 4.0074)
  line L4912 (29.2771, 4.0074) -> (29.465, 3.9734)
  line L4913 (29.465, 3.9734) -> (29.6661, 3.9326)
  line L4914 (29.6661, 3.9326) -> (29.8774, 3.8852)
  line L4915 (29.8774, 3.8852) -> (30.0989, 3.8305)
  line L4916 (30.0989, 3.8305) -> (30.3325, 3.7677)
  line L4917 (30.3325, 3.7677) -> (30.5755, 3.6968)
  line L4918 (30.5755, 3.6968) -> (30.7866, 3.6308)
  arc A153 (30.8688, 2.8495) -> (30.7866, 3.6308) centre (0, 0) ccw
  line L4919 (30.8688, 2.8495) -> (30.676, 2.741)
  point P0 (30.8688, 2.8495)
  point P1 (30.7866, 3.6308)
  point P2 (30.4018, 6.0605)
  point P3 (30.2385, 6.829)
  point P4 (29.6018, 9.2052)
  point P5 (29.359, 9.9523)
  point P6 (28.4774, 12.249)
  point P7 (28.1579, 12.9667)
  point P8 (27.041, 15.1586)
  point P9 (26.6482, 15.8389)
  point P10 (25.3084, 17.9021)
  point P11 (24.8466, 18.5377)
  point P12 (23.2985, 20.4495)
  point P13 (22.7728, 21.0333)
  point P14 (21.0333, 22.7728)
  point P15 (20.4495, 23.2985)
  point P16 (18.5377, 24.8466)
  point P17 (17.9021, 25.3084)
  point P18 (15.8389, 26.6482)
  point P19 (15.1586, 27.041)
  point P20 (12.9667, 28.1579)
  point P21 (12.249, 28.4774)
  point P22 (9.9523, 29.359)
  point P23 (9.2052, 29.6018)
  point P24 (6.0605, 30.4018)
  point P25 (3.6308, 30.7866)
  point P26 (2.8495, 30.8688)
  point P27 (0.3928, 30.9975)
  point P28 (-0.3928, 30.9975)
  point P29 (-2.8495, 30.8688)
  point P30 (-3.6308, 30.7866)
  point P31 (-6.0605, 30.4018)
  point P32 (-6.829, 30.2385)
  point P33 (-9.2052, 29.6018)
  point P34 (-9.9523, 29.359)
  point P35 (-12.249, 28.4774)
  point P36 (-12.9667, 28.1579)
  point P37 (-15.1586, 27.041)
  point P38 (-15.8389, 26.6482)
  point P39 (-17.9021, 25.3084)
  point P40 (-18.5377, 24.8466)
  point P41 (-20.4495, 23.2985)
  point P42 (-21.0333, 22.7728)
  point P43 (-22.7728, 21.0333)
  point P44 (-23.2985, 20.4495)
  point P45 (-24.8466, 18.5377)
  point P46 (-25.3084, 17.9021)
  point P47 (-26.6482, 15.8389)
  point P48 (-27.041, 15.1586)
  point P49 (-28.1579, 12.9667)
  point P50 (-28.4774, 12.249)
  point P51 (-29.359, 9.9523)
  point P52 (-29.6018, 9.2052)
  point P53 (-30.4018, 6.0605)
  point P54 (-30.7866, 3.6308)
  point P55 (-30.8688, 2.8495)
  point P56 (-30.9975, 0.3928)
  point P57 (-30.9975, -0.3928)
  point P58 (-30.8688, -2.8495)
  point P59 (-30.7866, -3.6308)
  point P60 (-30.4018, -6.0605)
  point P61 (-30.2385, -6.829)
  point P62 (-29.6018, -9.2052)
  point P63 (-29.359, -9.9523)
  point P64 (-28.4774, -12.249)
  point P65 (-28.1579, -12.9667)
  point P66 (-27.041, -15.1586)
  point P67 (-26.6482, -15.8389)
  point P68 (-25.3084, -17.9021)
  point P69 (-24.8466, -18.5377)
  point P70 (-23.2985, -20.4495)
  point P71 (-22.7728, -21.0333)
  point P72 (-21.0333, -22.7728)
  point P73 (-20.4495, -23.2985)
  point P74 (-18.5377, -24.8466)
  point P75 (-17.9021, -25.3084)
  point P76 (-15.8389, -26.6482)
  point P77 (-15.1586, -27.041)
  point P78 (-12.9667, -28.1579)
  point P79 (-12.249, -28.4774)
  point P80 (-9.9523, -29.359)
  point P81 (-9.2052, -29.6018)
  point P82 (-6.829, -30.2385)
  point P83 (-6.0605, -30.4018)
  point P84 (-3.6308, -30.7866)
  point P85 (-2.8495, -30.8688)
  point P86 (-0.3928, -30.9975)
  point P87 (0.3928, -30.9975)
  point P88 (2.8495, -30.8688)
  point P89 (3.6308, -30.7866)
  point P90 (6.0605, -30.4018)
  point P91 (6.829, -30.2385)
  point P92 (9.2052, -29.6018)
  point P93 (9.9523, -29.359)
  point P94 (12.249, -28.4774)
  point P95 (12.9667, -28.1579)
  point P96 (15.1586, -27.041)
  point P97 (15.8389, -26.6482)
  point P98 (17.9021, -25.3084)
  point P99 (18.5377, -24.8466)
  point P100 (20.4495, -23.2985)
  point P101 (21.0333, -22.7728)
  point P102 (22.7728, -21.0333)
  point P103 (23.2985, -20.4495)
  point P104 (24.8466, -18.5377)
  point P105 (25.3084, -17.9021)
  point P106 (26.6482, -15.8389)
  point P107 (27.041, -15.1586)
  point P108 (28.1579, -12.9667)
  point P109 (28.4774, -12.249)
  point P110 (29.359, -9.9523)
  point P111 (29.6018, -9.2052)
  point P112 (30.2385, -6.829)
  point P113 (30.4018, -6.0605)
  point P114 (30.7866, -3.6308)
  point P115 (30.8688, -2.8495)
  point P116 (30.9975, -0.3928)
  point P117 (30.9975, 0.3928)
  point P118 (30.4357, -4.7271)
  point P119 (30.8213, -5.2578)
  point P120 (32.9691, -7.1917)
  point P121 (33.5372, -7.5197)
  point P122 (36.286, -8.4128)
  point P123 (36.9384, -8.4814)
  point P124 (39.8127, -8.1793)
  point P125 (40.4366, -7.9766)
  point P126 (42.9396, -6.5315)
  point P127 (43.4271, -6.0925)
  point P128 (45.1259, -3.7543)
  point P129 (45.3927, -3.155)
  point P130 (45.9936, -0.328)
  point P131 (45.9936, 0.328)
  point P132 (45.3927, 3.155)
  point P133 (45.1259, 3.7543)
  point P134 (43.4271, 6.0925)
  point P135 (42.9396, 6.5315)
  point P136 (40.4366, 7.9766)
  point P137 (39.8127, 8.1793)
  point P138 (36.9384, 8.4814)
  point P139 (36.286, 8.4128)
  point P140 (33.5372, 7.5197)
  point P141 (32.9691, 7.1917)
  point P142 (30.8213, 5.2578)
  point P143 (30.4357, 4.7271)
  point P144 (29.2602, 2.0868)
  point P145 (29.1238, 1.4451)
  point P146 (29.1238, -1.4451)
  point P147 (29.2602, -2.0868)
  constraints: 9840 end point, 300 point on circle, 154 centre point
extrude "Extrusion1" add sketch "Sketch1" along normal blind 6.2 contours L827 L828 L829 L830 L831 L832 L833 L834 A20 L835 L836 L837 L838 L839 L840 L841 L842 L843 L844 L845 L846 L847 L848 L849 L850 L851 L852 L853 L854 L855 L856 L857 L858 L859 L860 L861 L862 A21 L863 L864 L865 L866 L867 L868 L869 L870 L871 L872 L873 L874 L875 L876 L877 L878 L879 L880 L881 L882 L883 L884 L885 L886 L887 L888 L889 L890 A22 L891 L892 L893 L894 L895 L896 L897 L898 L899 L900 L901 L902 L903 L904 L905 L906 L907 L908 L909 L910 L911 L912 L913 L914 L915 L916 L917 L918 A23 L919 L920 L921 L922 L923 L924 L925 L926 L927 L928 L929 L930 L931 L932 L933 L934 L935 L936 L937 L938 L939 L940 L941 L942 L943 L944 L945 L946 A24 L947 L948 L949 L950 L951 L952 L953 L954 L955 L956 L957 L958 L959 L960 L961 L962 L963 L964 L965 L966 L967 L968 L969 L970 L971 L972 L973 L974 A25 L975 L976 L977 L978 L979 L980 L981 L982 L983 L984 L985 L986 L987 L988 L989 L990 L991 L992 L993 L994 L995 L996 L997 L998 L999 L1000 L1001 L1002 A26 L1003 L1004 L1005 L1006 L1007 L1008 L1009 L1010 L1011 L1012 L1013 L1014 L1015 L1016 L1017 L1018 L1019 L1020 L1021 L1022 L1023 L1024 L1025 L1026 L1027 L1028 L1029 L1030 A27 L1031 L1032 L1033 L1034 L1035 L1036 L1037 L1038 L1039 L1040 L1041 L1042 L1043 L1044 L1045 L1046 L1047 L1048 L1049 L1050 L1051 L1052 L1053 L1054 L1055 L1056 L1057 L1058 A28 L1059 L1060 L1061 L1062 L1063 L1064 L1065 L1066 L1067 L1068 L1069 L1070 L1071 L1072 L1073 L1074 L1075 L1076 L1077 L1078 L1079 L1080 L1081 L1082 L1083 L1084 L1085 L1086 A29 L1087 L1088 L1089 L1090 L1091 L1092 L1093 L1094 L1095 L1096 L1097 L1098 L1099 L1100 L1101 L1102 L1103 L1104 L1105 L1106 L1107 L1108 L1109 L1110 L1111 L1112 L1113 L1114 A30 L1115 L1116 L1117 L1118 L1119 L1120 L1121 L1122 L1123 L1124 L1125 L1126 L1127 L1128 L1129 L1130 L1131 L1132 L1133 L1134 L1135 L1136 L1137 L1138 L1139 L1140 L1141 L1142 A31 L1143 L1144 L1145 L1146 L1147 L1148 L1149 L1150 L1151 L1152 L1153 L1154 L1155 L1156 L1157 L1158 L1159 L1160 L1161 L1162 L1163 L1164 L1165 L1166 L1167 L1168 L1169 L1170 A32 L1171 L1172 L1173 L1174 L1175 L1176 L1177 L1178 L1179 L1180 L1181 L1182 L1183 L1184 L1185 L1186 L1187 L1188 L1189 L1190 L1191 L1192 L1193 L1194 L1195 L1196 L1197 L1198 A33 L1199 L1200 L1201 L1202 L1203 L1204 L1205 L1206 L1207 L1208 L1209 L1210 L1211 L1212 L1213 L1214 L1215 L1216 L1217 L1218 L1219 L1220 L1221 L1222 L1223 L1224 L1225 L1226 A34 L1227 L1228 L1229 L1230 L1231 L1232 L1233 L1234 L1235 L1236 L1237 L1238 L1239 L1240 L1241 L1242 L1243 L1244 L1245 L1246 L1247 L1248 L1249 L1250 L1251 L1252 L1253 L1254 A35 L1255 L1256 L1257 L1258 L1259 L1260 L1261 L1262 L1263 L1264 L1265 L1266 L1267 L1268 L1269 L1270 L1271 L1272 L1273 L1274 L1275 L1276 L1277 L1278 L1279 L1280 L1281 L1282 A36 L1283 L1284 L1285 L1286 L1287 L1288 L1289 L1290 L1291 L1292 L1293 L1294 L1295 L1296 L1297 L1298 L1299 L1300 L1301 L1302 L1303 L1304 L1305 L1306 L1307 L1308 L1309 L1310 A37 L1311 L1312 L1313 L1314 L1315 L1316 L1317 L1318 L1319 L1320 L1321 L1322 L1323 L1324 L1325 L1326 L1327 L1328 L1329 L1330 L1331 L1332 L1333 L1334 L1335 L1336 L1337 L1338 A38 L1339 L1340 L1341 L1342 L1343 L1344 L1345 L1346 L1347 L1348 L1349 L1350 L1351 L1352 L1353 L1354 L1355 L1356 L1357 L1358 L1359 L1360 L1361 L1362 L1363 L1364 L1365 L1366 A39 L1367 L1368 L1369 L1370 L1371 L1372 L1373 L1374 L1375 L1376 L1377 L1378 L1379 L1380 L1381 L1382 L1383 L1384 L1385 L1386 L1387 L1388 L1389 L1390 L1391 L1392 L1393 L1394 A40 L1395 L1396 L1397 L1398 L1399 L1400 L1401 L1402 L1403 L1404 L1405 L1406 L1407 L1408 L1409 L1410 L1411 L1412 L1413 L1414 L1415 L1416 L1417 L1418 L1419 L1420 L1421 L1422 A41 L1423 L1424 L1425 L1426 L1427 L1428 L1429 L1430 L1431 L1432 L1433 L1434 L1435 L1436 L1437 L1438 L1439 L1440 L1441 L1442 L1443 L1444 L1445 L1446 L1447 L1448 L1449 L1450 A42 L1451 L1452 L1453 L1454 L1455 L1456 L1457 L1458 L1459 L1460 L1461 L1462 L1463 L1464 L1465 L1466 L1467 L1468 L1469 L1470 L1471 L1472 L1473 L1474 L1475 L1476 L1477 L1478 A43 L1479 L1480 L1481 L1482 L1483 L1484 L1485 L1486 L1487 L1488 L1489 L1490 L1491 L1492 L1493 L1494 L1495 L1496 L1497 L1498 L1499 L1500 L1501 L1502 L1503 L1504 L1505 L1506 A44 L1507 L1508 L1509 L1510 L1511 L1512 L1513 L1514 L1515 L1516 L1517 L1518 L1519 L1520 L1521 L1522 L1523 L1524 L1525 L1526 L1527 L1528 L1529 L1530 L1531 L1532 L1533 L1534 A45 L1535 L1536 L1537 L1538 L1539 L1540 L1541 L1542 L1543 L1544 L1545 L1546 L1547 L1548 L1549 L1550 L1551 L1552 L1553 L1554 L1555 L1556 L1557 L1558 L1559 L1560 L1561 L1562 A46 L1563 L1564 L1565 L1566 L1567 L1568 L1569 L1570 L1571 L1572 L1573 L1574 L1575 L1576 L1577 L1578 L1579 L1580 L1581 L1582 L1583 L1584 L1585 L1586 L1587 L1588 L1589 L1590 A47 L1591 L1592 L1593 L1594 L1595 L1596 L1597 L1598 L1599 L1600 L1601 L1602 L1603 L1604 L1605 L1606 L1607 L1608 L1609 L1610 L1611 L1612 L1613 L1614 L1615 L1616 L1617 L1618 A48 L1619 L1620 L1621 L1622 L1623 L1624 L1625 L1626 L1627 L1628 L1629 L1630 L1631 L1632 L1633 L1634 L1635 L1636 L1637 L1638 L1639 L1640 L1641 L1642 L1643 L1644 L1645 L1646 A49 L1647 L1648 L1649 L1650 L1651 L1652 L1653 L1654 L1655 L1656 L1657 L1658 L1659 L1660 L1661 L1662 L1663 L1664 L1665 L1666 L1667 L1668 L1669 L1670 L1671 L1672 L1673 L1674 A50 L1675 L1676 L1677 L1678 L1679 L1680 L1681 L1682 L1683 L1684 L1685 L1686 L1687 L1688 L1689 L1690 L1691 L1692 L1693 L1694 L1695 L1696 L1697 L1698 L1699 L1700 L1701 L1702 A51 L1703 L1704 L1705 L1706 L1707 L1708 L1709 L1710 L1711 L1712 L1713 L1714 L1715 L1716 L1717 L1718 L1719 L1720 L1721 L1722 L1723 L1724 L1725 L1726 L1727 L1728 L1729 L1730 A52 L1731 L1732 L1733 L1734 L1735 L1736 L1737 L1738 L1739 L1740 L1741 L1742 L1743 L1744 L1745 L1746 L1747 L1748 L1749 L1750 L1751 L1752 L1753 L1754 L1755 L1756 L1757 L1758 A53 L1759 L1760 L1761 L1762 L1763 L1764 L1765 L1766 L1767 L1768 L1769 L1770 L1771 L1772 L1773 L1774 L1775 L1776 L1777 L1778 L1779 L1780 L1781 L1782 L1783 L1784 L1785 L1786 A54 L1787 L1788 L1789 L1790 L1791 L1792 L1793 L1794 L1795 L1796 L1797 L1798 L1799 L1800 L1801 L1802 L1803 L1804 L1805 L1806 L1807 L1808 L1809 L1810 L1811 L1812 L1813 L1814 A55 L1815 L1816 L1817 L1818 L1819 L1820 L1821 L1822 L1823 L1824 L1825 L1826 L1827 L1828 L1829 L1830 L1831 L1832 L1833 L1834 L1835 L1836 L1837 L1838 L1839 L1840 L1841 L1842 A56 L1843 L1844 L1845 L1846 L1847 L1848 L1849 L1850 L1851 L1852 L1853 L1854 L1855 L1856 L1857 L1858 L1859 L1860 L1861 L1862 L1863 L1864 L1865 L1866 L1867 L1868 L1869 L1870 A57 L1871 L1872 L1873 L1874 L1875 L1876 L1877 L1878 L1879 L1880 L1881 L1882 L1883 L1884 L1885 L1886 L1887 L1888 L1889 L1890 L1891 L1892 L1893 L1894 L1895 L1896 L1897 L1898 A58 L1899 L1900 L1901 L1902 L1903 L1904 L1905 L1906 L1907 L1908 L1909 L1910 L1911 L1912 L1913 L1914 L1915 L1916 L1917 L1918 L1919 L1920 L1921 L1922 L1923 L1924 L1925 L1926 A59 L1927 L1928 L1929 L1930 L1931 L1932 L1933 L1934 L1935 L1936 L1937 L1938 L1939 L1940 L1941 L1942 L1943 L1944 L1945 L1946 L1947 L1948 L1949 L1950 L1951 L1952 L1953 L1954 A60 L1955 L1956 L1957 L1958 L1959 L1960 L1961 L1962 L1963 L1964 L1965 L1966 L1967 L1968 L1969 L1970 L1971 L1972 L1973 L1974 L1975 L1976 L1977 L1978 L1979 L1980 L1981 L1982 A61 L1983 L1984 L1985 L1986 L1987 L1988 L1989 L1990 L1991 L1992 L1993 L1994 L1995 L1996 L1997 L1998 L1999 L2000 L2001 L2002 L2003 L2004 L2005 L2006 L2007 L2008 L2009 L2010 A62 L2011 L2012 L2013 L2014 L2015 L2016 L2017 L2018 L2019 L2020 L2021 L2022 L2023 L2024 L2025 L2026 L2027 L2028 L2029 L2030 L2031 L2032 L2033 L2034 L2035 L2036 L2037 L2038 A63 L2039 L2040 L2041 L2042 L2043 L2044 L2045 L2046 L2047 L2048 L2049 L2050 L2051 L2052 L2053 L2054 L2055 L2056 L2057 L2058 L2059 L2060 L2061 L2062 L2063 L2064 L2065 L2066 A64 L2067 L2068 L2069 L2070 L2071 L2072 L2073 L2074 L2075 L2076 L2077 L2078 L2079 L2080 L2081 L2082 L2083 L2084 L2085 L2086 L2087 L2088 L2089 L2090 L2091 L2092 L2093 L2094 A65 L2095 L2096 L2097 L2098 L2099 L2100 L2101 L2102 L2103 L2104 L2105 L2106 L2107 L2108 L2109 L2110 L2111 L2112 L2113 L2114 L2115 L2116 L2117 L2118 L2119 L2120 L2121 L2122 A66 L2123 L2124 L2125 L2126 L2127 L2128 L2129 L2130 L2131 L2132 L2133 L2134 L2135 L2136 L2137 L2138 L2139 L2140 L2141 L2142 L2143 L2144 L2145 L2146 L2147 L2148 L2149 L2150 A67 L2151 L2152 L2153 L2154 L2155 L2156 L2157 L2158 L2159 L2160 L2161 L2162 L2163 L2164 L2165 L2166 L2167 L2168 L2169 L2170 L2171 L2172 L2173 L2174 L2175 L2176 L2177 L2178 A68 L2179 L2180 L2181 L2182 L2183 L2184 L2185 L2186 L2187 L2188 L2189 L2190 L2191 L2192 L2193 L2194 L2195 L2196 L2197 L2198 L2199 L2200 L2201 L2202 L2203 L2204 L2205 L2206 A69 L2207 L2208 L2209 L2210 L2211 L2212 L2213 L2214 L2215 L2216 L2217 L2218 L2219 L2220 L2221 L2222 L2223 L2224 L2225 L2226 L2227 L2228 L2229 L2230 L2231 L2232 L2233 L2234 A70 L2235 L2236 L2237 L2238 L2239 L2240 L2241 L2242 L2243 L2244 L2245 L2246 L2247 L2248 L2249 L2250 L2251 L2252 L2253 L2254 L2255 L2256 L2257 L2258 L2259 L2260 L2261 L2262 A71 L2263 L2264 L2265 L2266 L2267 L2268 L2269 L2270 L2271 L2272 L2273 L2274 L2275 L2276 L2277 L2278 L2279 L2280 L2281 L2282 L2283 L2284 L2285 L2286 L2287 L2288 L2289 L2290 A72 L2291 L2292 L2293 L2294 L2295 L2296 L2297 L2298 L2299 L2300 L2301 L2302 L2303 L2304 L2305 L2306 L2307 L2308 L2309 L2310 L2311 L2312 L2313 L2314 L2315 L2316 L2317 L2318 A73 L2319 L2320 L2321 L2322 L2323 L2324 L2325 L2326 L2327 L2328 L2329 L2330 L2331 L2332 L2333 L2334 L2335 L2336 L2337 L2338 L2339 L2340 L2341 L2342 L2343 L2344 L2345 L2346 A74 L2347 L2348 L2349 L2350 L2351 L2352 L2353 L2354 L2355 L2356 L2357 L2358 L2359 L2360 L2361 L2362 L2363 L2364 L2365 L2366 L2367 L2368 L2369 L2370 L2371 L2372 L2373 L2374 A75 L2375 L2376 L2377 L2378 L2379 L2380 L2381 L2382 L2383 L2384 L2385 L2386 L2387 L2388 L2389 L2390 L2391 L2392 L2393 L2394 L2395 L2396 L2397 L2398 L2399 L2400 L2401 L2402 A76 L2403 L2404 L2405 L2406 L2407 L2408 L2409 L2410 L2411 L2412 L2413 L2414 L2415 L2416 L2417 L2418 L2419 L2420 L2421 L2422 L2423 L2424 L2425 L2426 L2427 L2428 L2429 L2430 A77 L2431 L2432 L2433 L2434 L2435 L2436 L2437 L2438 L2439 L2440 L2441 L2442 L2443 L2444 L2445 L2446 L2447 L2448 L2449 L2450 L2451 L2452 L2453 L2454 L2455 L2456 L2457 L2458 A78 L2459 L780 L781 L782 L783 L784 L785 L786 L103 L787 L788 L789 L790 L791 L792 L793 L794 L795 L796 L797 L798 L799 L800 L801 L802 L803 L804 L805 L806 A19 L807 L808 L809 L810 L811 L812 L813 L814 L815 L816 L817 L818 L819 L820 L821 L822 L823 L824 L825 L826 L50
sketch "Sketch4" plane through (0, 0, 6.2) normal (0, 0, 1) x (1, 0, 0)
  line L0 (0, 0) -> (3.1, 0) construction
  circle A0 centre (0, 0) radius 2 construction
  line L1 (0, 0) -> (1.55, 2.6847) construction
  line L2 (0, 0) -> (-1.55, 2.6847) construction
  line L3 (0, 0) -> (-3.1, 0) construction
  line L4 (0, 0) -> (-1.55, -2.6847) construction
  line L5 (0, 0) -> (1.55, -2.6847) construction
  line L6 (-1.55, 2.6847) -> (1.55, 2.6847) construction
  line L7 (1.55, 2.6847) -> (3.1, 0) construction
  line L8 (3.1, 0) -> (1.55, -2.6847) construction
  line L9 (1.55, -2.6847) -> (-1.55, -2.6847) construction
  line L10 (-1.55, -2.6847) -> (-3.1, 0) construction
  line L11 (-3.1, 0) -> (-1.55, 2.6847) construction
  line L12 (3.6774, 0) -> (1.8387, 3.1847)
  line L13 (1.8387, 3.1847) -> (-1.8387, 3.1847)
  line L14 (-1.8387, 3.1847) -> (-3.6774, 0)
  line L15 (-3.6774, 0) -> (-1.8387, -3.1847)
  line L16 (-1.8387, -3.1847) -> (1.8387, -3.1847)
  line L17 (1.8387, -3.1847) -> (3.6774, 0)
  dimension "d20" = 3.1
  dimension "d23" = 360
  dimension "d34" = 0.5
  constraints: 36 end point, 6 parallel, 2 horizontal, 1 point on line, 24 other
  measures "d20" distance of L0.start L0.end
  measures "d34" distance between parallel lines of L7 L12
extrude "Extrusion7" cut sketch "Sketch4" against normal blind 10
body "Solid1"
